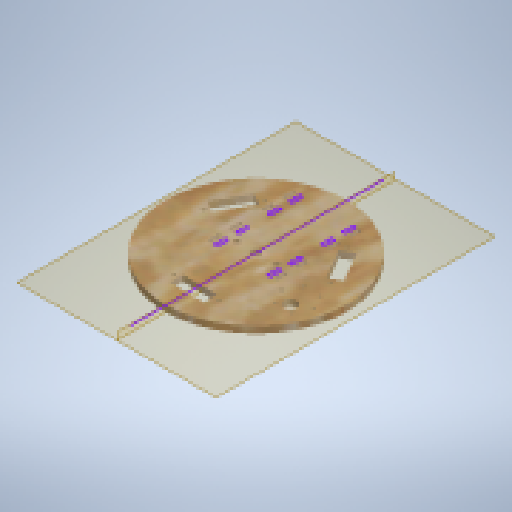
# Autodesk Inventor part: Fanerka
Saved by Autodesk Inventor 2023.2 (Build 272271030, 271C)
## iProperties
Created: 2023-12-24
Part Number: Fanerka
Material: Типовые
Document SubType Name: Modeling
Designer: Dell
Density: 1 g/cm^3
Appearance: По умолчанию
Mass: 125.819 g
Surface Area: 492.756 cm^2
Volume: 125.819 cm^3
Author: Dell
Autodesk Inventor part; units mm, degrees
ref_plane "XY Plane" through (0, 0, 0) normal (0, 0, 1) x (1, 0, 0)
sketch "Эскиз1" plane through (0, 0, 0) normal (0, 1, 0) x (-1, 0, 0)
  circle A0 centre (0, 0) radius 85
  circle A1 centre (0, 0) radius 4
  dimension "d0" = 170
  dimension "d15" = 8
  constraints: 2 centre point, 2 coincident
  measures "d0" diameter of A0
  measures "d15" diameter of A1
extrude "Выдавливание1" add sketch "Эскиз1" along normal blind 6
sketch "Эскиз2" plane through (0, 0, 0) normal (0, -1, 0) x (1, 0, 0)
  circle A0 centre (0, 0) radius 4 projected
  circle A1 centre (0, 0) radius 117.5181 construction
  line L0 (101.7737, 58.7591) -> (0, -117.5181) construction
  line L1 (0, -117.5181) -> (-101.7737, 58.7591) construction
  line L2 (-101.7737, 58.7591) -> (101.7737, 58.7591) construction
  line L3 (16.15, 64.9091) -> (-16.15, 64.9091)
  line L4 (-16.15, 64.9091) -> (-16.15, 52.6091)
  line L5 (-16.15, 52.6091) -> (16.15, 52.6091)
  line L6 (16.15, 52.6091) -> (16.15, 64.9091)
  line L7 (16.15, 64.9091) -> (-16.15, 52.6091) construction
  line L8 (-16.15, 64.9091) -> (16.15, 52.6091) construction
  line L9 (-16.15, 58.7591) -> (16.15, 58.7591) construction
  line L10 (-64.2879, -18.4682) -> (-48.1379, -46.4408)
  line L11 (-37.4858, -40.2908) -> (-53.6358, -12.3182)
  line L12 (-53.6358, -12.3182) -> (-64.2879, -18.4682)
  line L13 (-48.1379, -46.4408) -> (-37.4858, -40.2908)
  line L14 (-64.2879, -18.4682) -> (-37.4858, -40.2908) construction
  line L15 (-48.1379, -46.4408) -> (-53.6358, -12.3182) construction
  line L16 (48.1379, -46.4408) -> (64.2879, -18.4682)
  line L17 (53.6358, -12.3182) -> (37.4858, -40.2908)
  line L18 (37.4858, -40.2908) -> (48.1379, -46.4408)
  line L19 (64.2879, -18.4682) -> (53.6358, -12.3182)
  line L20 (48.1379, -46.4408) -> (53.6358, -12.3182) construction
  line L21 (64.2879, -18.4682) -> (37.4858, -40.2908) construction
  circle A2 centre (58.0718, 25.9871) radius 6
  circle A3 centre (18.6407, 0) radius 2.5
  circle A4 centre (-18.3593, 0) radius 2.5
  point P0 (0, 58.7591)
  point P1 (-58.9618, -15.3932)
  point P2 (-42.8118, -43.3658)
  point P3 (-50.8868, -29.3795)
  point P4 (42.8118, -43.3658)
  point P5 (58.9618, -15.3932)
  point P6 (50.8868, -29.3795)
  dimension "d16" = 32.3
  dimension "d17" = 12.3
  dimension "d20" = 360
  dimension "d25" = 12
  dimension "d26" = 5
  dimension "d27" = 5
  dimension "d28" = 37
  constraints: 44 end point, 5 midpoint, 3 centre point, 2 coincident, 2 parallel, 1 horizontal, 1 perpendicular, 1 point on line, 50 other
  measures "d16" distance of L5.end L4.end
  measures "d17" distance of L4.end L3.end
  measures "d25" diameter of A2
  measures "d26" diameter of A3
  measures "d27" diameter of A4
  measures "d28" distance of A3.centre A4.centre
extrude "Выдавливание3" cut sketch "Эскиз2" against normal blind 6 contours L6 L5 L4 L3 | L12 L11 L13 L10 | L18 L17 L19 L16 | A2 | A3 | A4
sketch "Эскиз3" plane through (0, 0, 0) normal (0, -1, 0) x (1, 0, 0)
  point P0 (0, 0)
sketch "Эскиз4" plane through (0, 0, 0) normal (0, -1, 0) x (1, 0, 0)
  point P0 (0, 0)
sketch "Эскиз5" plane through (0, 0, 0) normal (0, -1, 0) x (1, 0, 0)
  circle A0 centre (65.8248, 32.4068) radius 1.25 construction
  circle A1 centre (73.5684, 18.9798) radius 1.25 construction
  circle A2 centre (50.3248, 32.4142) radius 1.25 construction
  circle A3 centre (65.8121, 5.5601) radius 1.25 construction
  circle A4 centre (61.3843, 6.6933) radius 1.19 construction
  circle A5 centre (65.8121, 5.5601) radius 1.25 construction
  circle A6 centre (50.3121, 5.5674) radius 1.25 construction
  circle A7 centre (42.5684, 18.9944) radius 1.25 construction
  circle A8 centre (50.3248, 32.4142) radius 1.25 construction
  circle A9 centre (73.5684, 18.9798) radius 1.5
  circle A10 centre (65.8121, 5.5601) radius 1.5
  circle A11 centre (50.3121, 5.5674) radius 1.5
  circle A12 centre (42.5684, 18.9944) radius 1.5
  circle A13 centre (50.3248, 32.4142) radius 1.5
  circle A14 centre (65.8248, 32.4068) radius 1.5
  point P0 (0, 0)
  dimension "d29" = 3
  dimension "d30" = 3
  dimension "d31" = 3
  dimension "d32" = 3
  dimension "d33" = 3
  dimension "d34" = 3
  constraints: 6 centre point, 6 coincident
  measures "d29" diameter of A9
  measures "d30" diameter of A10
  measures "d31" diameter of A11
  measures "d32" diameter of A12
  measures "d33" diameter of A13
  measures "d34" diameter of A14
extrude "Выдавливание4" cut sketch "Эскиз5" against normal blind 10
sketch "Эскиз6" plane through (0, 0, 0) normal (0, -1, 0) x (1, 0, 0)
  circle A0 centre (-59.3361, -10.0795) radius 1.65 projected
  circle A1 centre (-38.3361, -46.4526) radius 1.65 projected
  circle A2 centre (38.6083, -46.4687) radius 1.65 projected
  circle A3 centre (59.6083, -10.0956) radius 1.65 projected
  circle A4 centre (21.15, 56.5482) radius 1.65 projected
  circle A5 centre (-20.85, 56.5482) radius 1.65 projected
  point P0 (0, 0)
extrude "Выдавливание5" cut sketch "Эскиз6" against normal blind 10
sketch "Эскиз7" plane through (0, 6, 0) normal (0, 1, 0) x (1, 0, 0)
  line L0 (0, 119) -> (0, -119)
  line L1 (23.4582, 57.0847) -> (26.4582, 57.0835)
  line L2 (23.4622, 67.0847) -> (23.4582, 57.0847)
  line L3 (26.4622, 67.0835) -> (23.4622, 67.0847)
  line L4 (26.4582, 57.0835) -> (26.4622, 67.0835)
  line L5 (23.4503, 37.0847) -> (26.4503, 37.0835)
  line L6 (23.4542, 47.0847) -> (23.4503, 37.0847)
  line L7 (26.4542, 47.0835) -> (23.4542, 47.0847)
  line L8 (26.4503, 37.0835) -> (26.4542, 47.0835)
  line L9 (-23.4776, 56.9868) -> (-26.4776, 56.9868)
  line L10 (-26.4776, 56.9868) -> (-26.4776, 66.9868)
  line L11 (-26.4776, 66.9868) -> (-23.4776, 66.9868)
  line L12 (-23.4776, 66.9868) -> (-23.4776, 56.9868)
  line L13 (-23.4776, 36.9868) -> (-26.4776, 36.9868)
  line L14 (-26.4776, 36.9868) -> (-26.4776, 46.9868)
  line L15 (-26.4776, 46.9868) -> (-23.4776, 46.9868)
  line L16 (-23.4776, 46.9868) -> (-23.4776, 36.9868)
  line L17 (-23.4776, 6.9868) -> (-26.4776, 6.9868)
  line L18 (-26.4776, 6.9868) -> (-26.4776, 16.9868)
  line L19 (-26.4776, 16.9868) -> (-23.4776, 16.9868)
  line L20 (-23.4776, 16.9868) -> (-23.4776, 6.9868)
  line L21 (23.4384, 7.0847) -> (26.4384, 7.0835)
  line L22 (23.4423, 17.0847) -> (23.4384, 7.0847)
  line L23 (26.4423, 17.0835) -> (23.4423, 17.0847)
  line L24 (26.4384, 7.0835) -> (26.4423, 17.0835)
  line L25 (23.4304, -12.9153) -> (26.4304, -12.9165)
  line L26 (23.4344, -2.9153) -> (23.4304, -12.9153)
  line L27 (26.4344, -2.9165) -> (23.4344, -2.9153)
  line L28 (26.4304, -12.9165) -> (26.4344, -2.9165)
  line L29 (-23.4776, -13.0132) -> (-26.4776, -13.0132)
  line L30 (-26.4776, -13.0132) -> (-26.4776, -3.0132)
  line L31 (-26.4776, -3.0132) -> (-23.4776, -3.0132)
  line L32 (-23.4776, -3.0132) -> (-23.4776, -13.0132)
  constraints: 66 end point, 4 perpendicular
sketch "Эскиз8" plane through (0, 0, 0) normal (0, -1, 0) x (1, 0, 0)
  line L0 (-32.5, -56.9877) -> (-32.5, -66.9877)
  line L1 (-29.5, -56.9877) -> (-32.5, -56.9877)
  line L2 (-29.5, -66.9877) -> (-29.5, -56.9877)
  line L3 (-32.5, -66.9877) -> (-29.5, -66.9877)
  line L4 (-29.5, -36.9877) -> (-32.5, -36.9877)
  line L5 (-32.5, -36.9877) -> (-32.5, -46.9877)
  line L6 (-32.5, -46.9877) -> (-29.5, -46.9877)
  line L7 (-29.5, -46.9877) -> (-29.5, -36.9877)
  line L8 (-29.5, -6.9877) -> (-32.5, -6.9877)
  line L9 (-32.5, -6.9877) -> (-32.5, -16.9877)
  line L10 (-32.5, -16.9877) -> (-29.5, -16.9877)
  line L11 (-29.5, -16.9877) -> (-29.5, -6.9877)
  line L12 (-29.5, 13.0123) -> (-32.5, 13.0123)
  line L13 (-32.5, 13.0123) -> (-32.5, 3.0123)
  line L14 (-32.5, 3.0123) -> (-29.5, 3.0123)
  line L15 (-29.5, 3.0123) -> (-29.5, 13.0123)
  line L16 (29.5, 13.0123) -> (32.5, 13.0123)
  line L17 (29.5, 3.0123) -> (29.5, 13.0123)
  line L18 (32.5, 3.0123) -> (29.5, 3.0123)
  line L19 (32.5, 13.0123) -> (32.5, 3.0123)
  line L20 (29.5, -6.9877) -> (32.5, -6.9877)
  line L21 (29.5, -16.9877) -> (29.5, -6.9877)
  line L22 (32.5, -16.9877) -> (29.5, -16.9877)
  line L23 (32.5, -6.9877) -> (32.5, -16.9877)
  line L24 (29.5, -36.9877) -> (32.5, -36.9877)
  line L25 (29.5, -46.9877) -> (29.5, -36.9877)
  line L26 (32.5, -46.9877) -> (29.5, -46.9877)
  line L27 (32.5, -36.9877) -> (32.5, -46.9877)
  line L28 (29.5, -56.9877) -> (32.5, -56.9877)
  line L29 (29.5, -66.9877) -> (29.5, -56.9877)
  line L30 (32.5, -66.9877) -> (29.5, -66.9877)
  line L31 (32.5, -56.9877) -> (32.5, -66.9877)
  constraints: 64 end point
extrude "Выдавливание7" cut sketch "Эскиз8" against normal up to surface (6 mm away)
sketch "Эскиз9" plane through (0, 6, 0) normal (0, 1, 0) x (1, 0, 0)
  line L0 (-29.5, 6.9877) -> (-32.5, 6.9877) projected
  line L1 (-32.5, -3.0123) -> (-29.5, -3.0123) projected
  line L2 (-29.5, 56.9877) -> (-32.5, 56.9877) projected
  line L3 (-32.5, 46.9877) -> (-29.5, 46.9877) projected
  line L4 (32.5, 56.9877) -> (29.5, 56.9877) projected
  line L5 (29.5, 46.9877) -> (32.5, 46.9877) projected
  line L6 (32.5, 6.9877) -> (29.5, 6.9877) projected
  line L7 (29.5, -3.0123) -> (32.5, -3.0123) projected
  line L8 (-29.5, 46.9877) -> (-32.5, 46.9877) projected
  line L9 (-31, 46.9877) -> (-31, 56.9877) construction
  line L10 (-32.5, 56.9877) -> (-29.5, 56.9877) projected
  line L11 (31, 56.9877) -> (31, 46.9877) construction
  line L12 (32.5, 46.9877) -> (29.5, 46.9877) projected
  line L13 (29.5, 6.9877) -> (32.5, 6.9877) projected
  line L14 (31, 6.9877) -> (31, -3.0123) construction
  line L15 (32.5, -3.0123) -> (29.5, -3.0123) projected
  line L16 (-32.5, 6.9877) -> (-29.5, 6.9877) projected
  line L17 (-31, 6.9877) -> (-31, -3.0123) construction
  circle A0 centre (-31, 51.9877) radius 1.5
  circle A1 centre (31, 51.9877) radius 1.5
  circle A2 centre (31, 1.9877) radius 1.5
  circle A3 centre (-31, 1.9877) radius 1.5
  point P0 (0, 0)
  dimension "d54" = 3
  constraints: 12 midpoint, 8 end point, 4 centre point, 3 equal radius, 3 perpendicular
  measures "d54" diameter of A0
extrude "Выдавливание8" cut sketch "Эскиз9" against normal up to surface (6 mm away)
